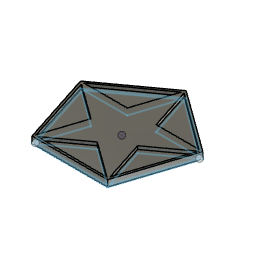
3D Plancha 2 (Autodesk Fusion 360 design; units mm, degrees)
Autodesk Fusion 360 part; units mm, degrees
sketch "Boceto1" plane through (0, 0, 0) normal (0, 0, 1) x (1, 0, 0)
  line L0 (0, 10) -> (-9.5106, 3.0902)
  line L1 (-9.5106, 3.0902) -> (-5.8779, -8.0902)
  line L2 (-5.8779, -8.0902) -> (5.8779, -8.0902)
  line L3 (5.8779, -8.0902) -> (9.5106, 3.0902)
  line L4 (9.5106, 3.0902) -> (0, 10)
  line L5 (-9.0281, 2.7396) -> (-5.6882, -7.738)
  line L6 (-5.3954, -7.7396) -> (5.4788, -7.8003)
  line L7 (5.6936, -7.523) -> (9.1501, 2.9168)
  line L8 (8.9142, 3.0902) -> (0.1524, 9.5309)
  line L9 (-0.1843, 9.4328) -> (-9.0173, 3.0902)
  line L10 (-9.0173, 3.0902) -> (-2.2451, 3.0902)
  line L11 (2.2451, 3.0902) -> (8.9142, 3.0902)
  line L12 (-9.0281, 2.7396) -> (-3.6327, -1.1803)
  line L13 (0, -3.8197) -> (5.4788, -7.8003)
  line L14 (9.1115, 2.8003) -> (3.6327, -1.1803)
  line L15 (0, -3.8197) -> (-5.3954, -7.7396)
  line L16 (-0.1843, 9.4328) -> (-2.2451, 3.0902)
  line L17 (-3.6327, -1.1803) -> (-5.7254, -7.6211)
  line L18 (0.1524, 9.5309) -> (2.2451, 3.0902)
  line L19 (3.6327, -1.1803) -> (5.6936, -7.523)
  constraint horizontal L10
  constraint coincident L5 L17.end
  constraint coincident L7 L14.start
  constraint collinear L10 L11
  constraint coincident L12.end L16
  constraint coincident L13.start L14
  constraint collinear L12 L13
  constraint coincident L14.end L18
  constraint collinear L14 L15
  constraint collinear L16 L17
  constraint collinear L18 L19
extrude "Extruir1" add sketch "Boceto1" along normal blind 0.5 contours L5 L12 L17 | L6 L13 L15 | L7 L14 L19 | L8 L11 L18 | L9 L10 L16 makes body 1 at (0.0278, -6.4532, 0) makes body 2 at (-6.1287, -2.0206, 0) makes body 3 at (6.1459, -1.9677, 0) makes body 4 at (-3.8156, 5.2044, 0) makes body 5 at (3.7706, 5.2371, 0)
extrude "Extruir2" add sketch "Boceto1" along normal blind 1 bodies 1 2 3 4 5
